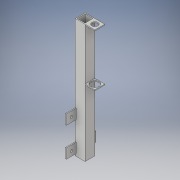
# Autodesk Inventor part: Mount for Control Panel
Saved by Autodesk Inventor 2017 (Build 210142000, 142)
## iProperties
Created: 2020-02-25
Part Number: Mount for Control Panel
Material: Generic
Document SubType Name: Modeling
Designer: S332862739
Density: 1 g/cm^3
Appearance: Default
Author: S332862739
Autodesk Inventor part; units mm, degrees
ref_plane "YZ Plane" through (0, 0, 0) normal (1, 0, 0) x (0, 1, 0)
ref_plane "XZ Plane" through (0, 0, 0) normal (0, 1, 0) x (-1, 0, 0)
ref_plane "XY Plane" through (0, 0, 0) normal (0, 0, 1) x (1, 0, 0)
sketch "Sketch1" plane through (0, 0, 0) normal (0, 1, 0) x (-1, 0, 0)
  line L0 (0, 0) -> (25.4, 0)
  line L1 (25.4, 0) -> (25.4, -25.4)
  line L2 (25.4, -25.4) -> (0, -25.4)
  line L3 (0, -25.4) -> (0, 0)
  dimension "d0" = 25.4
  dimension "d1" = 25.4
  constraints: 8 end point, 2 parallel, 1 horizontal, 1 perpendicular
  measures "d0" distance of L1.end L2.end
  measures "d1" distance of L0.end L1.end
extrude "Extrusion1" add sketch "Sketch1" along normal blind 307.975
sketch "Sketch2" plane through (0, 307.975, 0) normal (0, 1, 0) x (1, 0, 0)
  line L0 (-22.86, 2.54) -> (-2.54, 2.54)
  line L1 (-2.54, 2.54) -> (-2.54, 22.86)
  line L2 (-2.54, 22.86) -> (-22.86, 22.86)
  line L3 (-22.86, 22.86) -> (-22.86, 2.54)
  line L4 (-25.4, 0) -> (0, 0) projected
  line L5 (-25.4, 25.4) -> (-25.4, 0) projected
  dimension "d4" = 20.32
  dimension "d5" = 20.32
  dimension "d6" = 2.54
  dimension "d7" = 2.54
  constraints: 8 end point, 2 parallel, 1 horizontal, 1 perpendicular
  measures "d4" distance of L2.end L1.end
  measures "d5" distance of L1.end L0.end
  measures "d6" distance between parallel lines of L0 L4
  measures "d7" distance between parallel lines of L3 L5
extrude "Extrusion2" cut sketch "Sketch2" against normal blind 307.975
sketch "Sketch3" plane through (0, 0, 0) normal (1, 0, 0) x (0, 0, -1)
  line L0 (0, 0) -> (0, 307.975) projected
  line L1 (0, 307.975) -> (25.4, 307.975)
  line L2 (25.4, 307.975) -> (25.4, 305.435)
  line L3 (25.4, 305.435) -> (0, 305.435)
  line L4 (0, 305.435) -> (0, 307.975)
  dimension "d10" = 25.4
  dimension "d11" = 2.54
  constraints: 8 end point, 2 parallel, 1 horizontal, 1 perpendicular
  measures "d10" distance of L2.end L3.end
  measures "d11" distance of L1.end L2.end
extrude "Extrusion3" add sketch "Sketch3" along normal blind 25.4
sketch "Sketch4" plane through (0, 307.975, 0) normal (0, 1, 0) x (1, 0, 0)
  circle A0 centre (12.7, 12.7) radius 7.9121
  line L0 (-25.4, 0) -> (25.4, 0) projected
  line L1 (25.4, 25.4) -> (25.4, 0) projected
  point P0 (0, 0)
  dimension "d14" = 15.8242
  dimension "d15" = 12.7
  dimension "d16" = 12.7
  constraints: 1 centre point
  measures "d14" diameter of A0
  measures "d15" distance from line of A0.centre L0
  measures "d16" distance from line of L1 A0.centre
extrude "Extrusion4" cut sketch "Sketch4" against normal blind 25.4
sketch "Sketch5" plane through (0, 0, 0) normal (1, 0, 0) x (0, 0, -1)
  line L0 (0, 173.8561) -> (25.4, 173.8561)
  line L1 (25.4, 173.8561) -> (25.4, 171.3161)
  line L2 (25.4, 171.3161) -> (0, 171.3161)
  line L3 (0, 171.3161) -> (0, 173.8561)
  point P0 (0, 0)
  dimension "d19" = 25.4
  dimension "d20" = 2.54
  constraints: 8 end point, 2 parallel, 1 horizontal, 1 perpendicular
  measures "d19" distance of L1.end L2.end
  measures "d20" distance of L0.end L1.end
extrude "Extrusion5" add sketch "Sketch5" along normal blind 25.4
sketch "Sketch6" plane through (0, 171.3161, -25.4) normal (0, -1, 0) x (1, 0, 0)
  circle A0 centre (12.7, 12.7) radius 10.9601
  line L0 (0, 0) -> (25.4, 0) projected
  line L1 (25.4, 25.4) -> (25.4, 0) projected
  point P0 (0, 25.4)
  dimension "d23" = 21.9202
  dimension "d24" = 12.7
  dimension "d25" = 1.7399
  constraints: 1 centre point
  measures "d23" diameter of A0
  measures "d24" distance from line of L0 A0.centre
  measures "d25" distance edge to line of A0 L1
extrude "Extrusion6" cut sketch "Sketch6" against normal blind 25.4
sketch "Sketch7" plane through (-25.4, 0, 0) normal (0, 0, 1) x (1, 0, 0)
  line L0 (0, 0) -> (0, 307.975) projected
  line L1 (0, 31.75) -> (2.54, 31.75)
  line L2 (2.54, 31.75) -> (2.54, 6.35)
  line L3 (2.54, 6.35) -> (0, 6.35)
  line L4 (0, 6.35) -> (0, 31.75)
  line L5 (25.4, 0) -> (0, 0) projected
  line L6 (0, 0) -> (0, 307.975) projected
  line L7 (2.54, 307.975) -> (2.54, 0) projected
  line L8 (0, 82.55) -> (2.54, 82.55)
  line L9 (2.54, 82.55) -> (2.54, 107.95)
  line L10 (2.54, 107.95) -> (0, 107.95)
  line L11 (0, 107.95) -> (0, 82.55)
  dimension "d28" = 2.54
  dimension "d30" = 6.35
  dimension "d48" = 25.4
  dimension "d49" = 25.4
  dimension "d50" = 50.8
  constraints: 16 end point, 4 parallel, 3 point on line, 2 horizontal, 2 perpendicular
  measures "d28" distance of L2.end L3.end
  measures "d30" distance between parallel lines of L5 L3
  measures "d48" distance of L1.end L2.end
  measures "d49" distance of L9.end L8.end
  measures "d50" distance between parallel lines of L1 L8
sketch "Sketch8" plane through (0, 0, -25.4) normal (0, 0, -1) x (-1, 0, 0)
  line L0 (25.4, 0) -> (25.4, 307.975) projected
  line L1 (25.4, 31.75) -> (22.86, 31.75)
  line L2 (22.86, 31.75) -> (22.86, 6.35)
  line L3 (22.86, 6.35) -> (25.4, 6.35)
  line L4 (25.4, 6.35) -> (25.4, 31.75)
  line L5 (25.4, 0) -> (0, 0) projected
  dimension "d33" = 2.54
  dimension "d34" = 25.4
  dimension "d35" = 31.75
  constraints: 8 end point, 2 parallel, 1 horizontal, 1 perpendicular, 1 point on line
  measures "d33" distance of L3.end L2.end
  measures "d34" distance of L2.end L1.end
  measures "d35" distance between parallel lines of L5 L1
extrude "Extrusion8" add sketch "Sketch8" along normal blind 25.4
sketch "Sketch10" plane through (-22.86, 6.35, -25.4) normal (1, 0, 0) x (0, 0, -1)
  circle A0 centre (12.7, 12.7) radius 3.175
  line L0 (0, 0) -> (25.4, 0) projected
  line L1 (0, -6.35) -> (0, 164.9661) projected
  point P0 (-25.4, -6.35)
  dimension "d43" = 6.35
  dimension "d44" = 12.7
  dimension "d45" = 12.7
  constraints: 1 centre point
  measures "d43" diameter of A0
  measures "d44" distance from line of L0 A0.centre
  measures "d45" distance from line of A0.centre L1
extrude "Extrusion10" cut sketch "Sketch10" against normal blind 25.4
extrude "Extrusion11" add sketch "Sketch7" along normal blind 25.4 contours L0 L1 L2 L3 | L0 L10 L7 L8
sketch "Sketch11" plane through (-22.86, 82.55, 0) normal (1, 0, 0) x (0, 0, -1)
  circle A0 centre (-12.7, -63.5) radius 3.175
  line L0 (0, -50.8) -> (-25.4, -50.8) projected
  line L1 (-12.7, -50.8) -> (-12.7, -63.5) construction
  line L2 (-12.7, -63.5) -> (-25.4, -63.5) construction
  circle A1 centre (-12.7, 12.7) radius 3.175
  line L3 (-12.7, 12.7) -> (-12.7, 25.4) construction
  line L4 (0, 25.4) -> (-25.4, 25.4) projected
  line L5 (-12.7, 12.7) -> (-25.4, 12.7) construction
  point P0 (0, -82.55)
  dimension "d53" = 6.35
  dimension "d54" = 12.7
  dimension "d55" = 6.35
  dimension "d56" = 12.7
  constraints: 8 end point, 4 perpendicular, 2 centre point, 2 midpoint, 1 horizontal, 1 vertical
  measures "d53" diameter of A0
  measures "d54" distance of L1.start L1.end
  measures "d55" diameter of A1
  measures "d56" distance of L3.start L3.end
extrude "Extrusion12" cut sketch "Sketch11" against normal blind 25.4
body "Solid1"
